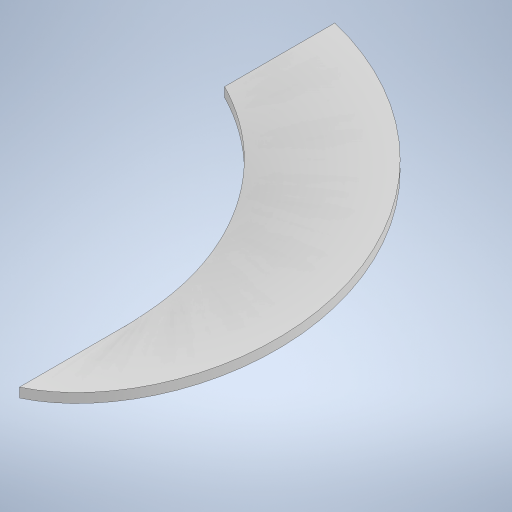
# Autodesk Inventor part: Espira_01_Parcial
Saved by Autodesk Inventor 2024 (Build 280153000, 153)
## iProperties
Created: 2026-01-07
Part Number: Espira_01_Parcial
Material: Generic
Document SubType Name: Modeling
Designer: eduso
Density: 1 g/cm^3
Appearance: Default
Paso_Espira_01: 200,000 mm
ø_Ext_Espira_01: 200,000 mm
ø_Int_Espira_01: 60,300 mm
Espesor_Espira_01: 6,000 mm
Author: eduso
Autodesk Inventor part; units mm, degrees
ref_plane "YZ Plane" through (0, 0, 0) normal (1, 0, 0) x (0, 1, 0)
ref_plane "XY Plane" through (0, 0, 0) normal (0, 0, 1) x (1, 0, 0)
sketch "Sketch1" plane through (0, 0, 0) normal (0, 1, 0) x (-1, 0, 0)
  circle A0 centre (0, 0) radius 30.15 construction
  line L0 (0, 0) -> (0, 30.15) construction
  dimension "d0" = 60.3
  constraints: 2 end point, 1 coincident, 1 vertical, 1 vertical alignment, 2 other
ref_plane "Work Plane1" through (0, 6, 0) normal (0, 1, 0) x (-1, 0, 0)
sketch "Sketch2" plane through (0, 6, 0) normal (0, 1, 0) x (-1, 0, 0)
  circle A0 centre (0, 0) radius 100 construction
  line L0 (0, 0) -> (0, 100) construction
  dimension "d2" = 200
  constraints: 2 end point, 1 coincident, 1 vertical, 1 vertical alignment, 2 other
sketch "Sketch3" plane through (0, 0, 0) normal (1, 0, 0) x (0, 1, 0)
  line L0 (0, 30.1075) -> (6.003, 30.1075)
  line L1 (6.003, 30.1075) -> (6.003, 100.0036)
  line L2 (6.003, 100.0036) -> (0, 100.0036)
  line L3 (0, 100.0036) -> (0, 30.1075)
  line L4 (0, 0) -> (200, 0) construction
  dimension "d3" = 200
  constraints: 10 end point, 2 horizontal, 2 parallel, 1 perpendicular
  measures "d3" distance of L4.start L4.end
coil "Coil1" sketch "Sketch3" operation add axis through (0, 0, 0) along (0, 1, 0) pitch 200 turns 0.5 hand right
equation "\"d0\" = ø_Int_Espira_01"
equation "\"d2\" = ø_Ext_Espira_01"
equation "\"d6\" = Ang_parcial"
equation "\"ø_Ext_Espira_01\" = 200"
equation "\"ø_Int_Espira_01\" = 60.3"
equation "\"Espesor_Espira_01\" = 6"
equation "\"d1\" = Espesor_Espira_01"
equation "\"L_parcial\" = 225"
equation "\"Ang_parcial\" = 0.5"
body "Solid1"
